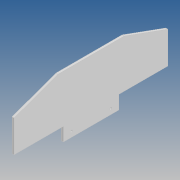
# Autodesk Inventor part: KB33-046-004-007 - Центральная левая боковая пластина
Saved by Autodesk Inventor 2020 (Build 240168000, 168)
## iProperties
Created: 2021-06-25
Part Number: KB33-046-004-007 - Центральная левая боковая пластина
Material: Типовые
Document SubType Name: Modeling
Designer: Петров Иван
Density: 1 g/cm^3
Appearance: По умолчанию
Mass: 104.886 g
Surface Area: 555.871 cm^2
Volume: 104.886 cm^3
Author: Петров Иван
Autodesk Inventor part; units mm, degrees
ref_plane "YZ Plane" through (0, 0, 0) normal (1, 0, 0) x (0, 1, 0)
ref_plane "XZ Plane" through (0, 0, 0) normal (0, 1, 0) x (-1, 0, 0)
ref_plane "XY Plane" through (0, 0, 0) normal (0, 0, 1) x (1, 0, 0)
sketch "Эскиз1" plane through (0, 0, 0) normal (1, 0, 0) x (0, 1, 0)
  line L0 (-10.528, 98.8876) -> (15, 98.8876)
  line L1 (15, 98.8876) -> (15, -5.1124)
  line L2 (15, -5.1124) -> (-10.528, -5.1124)
  line L3 (-10.528, -5.1124) -> (-10.528, 98.8876)
  point P0 (0, 0)
  dimension "d0" = 25.528
  dimension "d1" = 104
  constraints: 8 end point, 2 parallel, 1 horizontal, 1 perpendicular
  measures "d0" distance of L1.end L2.end
  measures "d1" distance of L0.end L1.end
extrude "Выдавливание1" add sketch "Эскиз1" along normal blind 4
sketch "Эскиз2" plane through (4, 0, 0) normal (1, 0, 0) x (0, 0, -1)
  circle A0 centre (-9.8876, -0.528) radius 2 projected
  circle A1 centre (-83.8876, -0.528) radius 2 projected
  point P0 (0, 0)
extrude "Выдавливание2" cut sketch "Эскиз2" against normal blind 4
sketch "Эскиз3" plane through (4, 0, 0) normal (1, 0, 0) x (0, 0, -1)
  line L0 (-191.6906, 75) -> (97.9154, 75)
  line L1 (97.9154, 75) -> (97.9154, 15)
  line L2 (97.9154, 15) -> (-191.6906, 15)
  line L3 (-191.6906, 15) -> (-191.6906, 75)
  line L4 (-98.8876, 15) -> (-98.8876, -10.528) projected
  line L5 (5.1124, -10.528) -> (5.1124, 15) projected
  point P0 (0, 0)
  dimension "d6" = 92.803
  dimension "d7" = 92.803
  dimension "d8" = 60
  constraints: 8 end point, 2 parallel, 1 horizontal, 1 perpendicular, 1 point on line
  measures "d6" distance between parallel lines of L3 L4
  measures "d7" distance between parallel lines of L1 L5
  measures "d8" distance between parallel lines of L2 L0
extrude "Выдавливание3" add sketch "Эскиз3" against normal blind 4
sketch "Эскиз4" plane through (4, 0, 0) normal (1, 0, 0) x (0, 0, -1)
  line L0 (-191.6906, 75) -> (97.9154, 75) projected
  line L1 (-191.6906, 75) -> (-109.2663, 105)
  line L2 (-109.2663, 105) -> (15.491, 105)
  line L3 (15.491, 105) -> (97.9154, 75)
  line L4 (97.9154, 75) -> (-191.6906, 75) projected
  line L5 (-98.8876, -10.528) -> (5.1124, -10.528) projected
  line L6 (-46.8876, -10.528) -> (-46.8876, 5.327)
  point P0 (0, 0)
  dimension "d11" = 30
  dimension "d12" = 20
  constraints: 8 end point, 1 midpoint, 1 parallel, 1 vertical, 1 other
  measures "d11" distance between parallel lines of L0 L2
  measures "d12" angle of L0 L3
extrude "Выдавливание4" add sketch "Эскиз4" against normal blind 4
equation "\"d7\" = d6"
